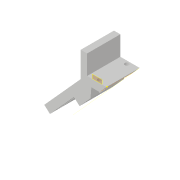
# Autodesk Inventor part: arm stop 48 degree bottom half
Saved by Autodesk Inventor 2018 (Build 220112000, 112)
## iProperties
Created: 2018-12-28
Part Number: arm stop 48 degree bottom half
Material: Generic
Document SubType Name: Modeling
Designer: ball
Density: 1 g/cm^3
Appearance: Default
Author: ball
Autodesk Inventor part; units mm, degrees
ref_plane "YZ Plane" through (0, 0, 0) normal (1, 0, 0) x (0, 1, 0)
ref_plane "XZ Plane" through (0, 0, 0) normal (0, 1, 0) x (-1, 0, 0)
ref_plane "Work Plane1" through (0, 0, 0) normal (0, 0, 1) x (1, 0, 0)
sketch "Sketch1" plane through (0, 0, 0) normal (0, 0, 1) x (1, 0, 0)
  line L0 (4.129202, -9.5377) -> (6.406797, -9.5377) construction
  line L1 (9.525, -8.41296) -> (9.525, -7.435497) construction
  line L2 (-6.406797, 9.5123) -> (-4.129202, 9.5123) construction
  line L3 (-9.525, 4.116502) -> (-9.525, 6.394097) construction
  line L4 (9.314549, -9.373063) -> (-73.965447, -101.864868) construction
  line L5 (9.166309, -9.5377) -> (-73.965447, -101.864868)
  line L6 (-73.965447, -101.864868) -> (-85.121243, -91.820144)
  line L7 (6.33881, 9.756536) -> (-85.121243, -91.820144) construction
  line L8 (9.166309, -9.5377) -> (-9.997679, -9.5377)
  line L9 (-9.997679, -9.5377) -> (-9.997679, 9.756536)
  line L10 (-9.997679, 9.756536) -> (-16.347679, 9.756536)
  line L11 (-16.347679, 9.756536) -> (-16.347679, -15.439362)
  line L12 (-16.347679, -15.439362) -> (-85.121243, -91.820144)
  point P0 (0, 0)
  dimension "d0" = 124.46
  dimension "d1" = 48
  dimension "d5" = 6.35
  constraints: 26 end point, 4 point on line, 3 horizontal, 3 perpendicular, 2 collinear, 2 vertical, 1 parallel, 8 other
  measures "d0" distance of L4.start L4.end
  measures "d1" angle of L0 L4
  measures "d5" distance of L9.end L10.end
ref_plane "Work Plane2" through (-4.445, -9.144, -33.02) normal (0, 0, -1) x (0, 1, 0)
extrude "Extrusion1" add sketch "Sketch1" against normal up to surface (33.02 mm away)
sketch "Sketch2" plane through (-73.965447, -101.864868, -33.02) normal (-0.6691306, -0.7431448, 0) x (0.7431448, -0.6691306, 0)
  line L0 (0, 33.02) -> (0, 0)
  line L1 (-15.011605, 33.02) -> (-15.011605, 0)
  line L2 (0, 0) -> (-15.011605, 0)
  line L3 (-15.011605, 0) -> (-15.011605, 26.67)
  line L4 (-15.011605, 26.67) -> (0, 26.67)
  line L5 (0, 26.67) -> (0, 0)
  line L6 (-15.011605, 33.02) -> (0, 33.02)
  point P0 (-13.193862, 33.02)
  dimension "d19" = 6.35
  constraints: 8 end point, 2 parallel, 1 horizontal, 1 perpendicular, 1 point on line
  measures "d19" distance between parallel lines of L6 L4
extrude "Extrusion2" cut sketch "Sketch2" against normal blind 25.4 contours L0 L2 L1 L4
sketch "Sketch3" plane through (-73.965447, -101.864868, -6.35) normal (0, 0, -1) x (-0.7431448, 0.6691306, 0)
  line L0 (19.8882, 12.0904) -> (19.8882, 3.175) construction
  line L1 (0, 25.4) -> (15.011605, 25.4) construction
  line L2 (15.011605, 0) -> (0, 0) construction
  line L3 (0, 0) -> (19.8882, 0) construction
  line L4 (19.8882, 0) -> (19.8882, 25.4) construction
  line L5 (19.8882, 25.4) -> (0, 25.4) construction
  line L6 (0, 25.4) -> (0, 0) construction
  line L7 (15.011605, 0) -> (19.8882, 0)
  line L8 (19.8882, 0) -> (19.8882, 25.4)
  line L9 (19.8882, 25.4) -> (15.011605, 25.4)
  line L10 (15.011605, 25.4) -> (15.011605, 0)
  point P0 (13.193862, 125.192894)
  constraints: 18 end point, 4 parallel, 2 horizontal, 2 perpendicular, 1 vertical, 2 other
extrude "Extrusion3" add sketch "Sketch3" against normal up to surface (6.35 mm away)
sketch "Sketch4" plane through (0, 0, 0) normal (0, 0, 1) x (1, 0, 0)
  line L0 (-88.74526, -88.557064) -> (-71.749342, -69.681186) construction
  line L1 (-73.965447, -101.864868) -> (9.166309, -9.5377) construction
  line L2 (-74.314967, -94.50927) -> (-67.5166, -86.958918) construction
  line L3 (-73.965447, -101.864868) -> (-56.969529, -82.988989) construction
  line L4 (-73.965447, -101.864868) -> (-88.74526, -88.557064) construction
  line L5 (-81.390199, -88.138702) -> (-74.591832, -80.588351) construction
  line L6 (-74.314967, -94.50927) -> (-67.5166, -86.958918) construction
  line L7 (-73.144662, -95.563017) -> (-66.346296, -88.012665)
  line L8 (-68.686904, -85.905171) -> (-75.485271, -93.455523)
  arc A0 (-75.485271, -93.455523) -> (-73.144662, -95.563017) centre (-74.314967, -94.50927) ccw
  arc A1 (-66.346296, -88.012665) -> (-68.686904, -85.905171) centre (-67.5166, -86.958918) ccw
  line L9 (-81.390199, -88.138702) -> (-74.591832, -80.588351) construction
  line L10 (-80.219894, -89.192449) -> (-73.421527, -81.642098)
  line L11 (-75.762136, -79.534604) -> (-82.560503, -87.084955)
  arc A2 (-82.560503, -87.084955) -> (-80.219894, -89.192449) centre (-81.390199, -88.138702) ccw
  arc A3 (-73.421527, -81.642098) -> (-75.762136, -79.534604) centre (-74.591832, -80.588351) ccw
  point P0 (0, 0)
  point P1 (-70.915783, -90.734094)
  point P2 (-77.991015, -84.363527)
  dimension "d37" = 10.16
  dimension "d38" = 5.1816
  dimension "d39" = 5.2324
  dimension "d40" = 9.52066
  dimension "d41" = 3.1496
  dimension "d42" = 3.1496
  constraints: 20 end point, 8 point on circle, 8 tangent, 4 centre point, 4 parallel, 2 collinear, 2 midpoint
  measures "d37" distance of L2.start L2.end
  measures "d38" distance between parallel lines of L1 L2
  measures "d39" distance from line of L2.start L4
  measures "d40" distance between parallel lines of L2 L5
  measures "d41" diameter of A1
  measures "d42" diameter of A3
extrude "Extrusion4" cut sketch "Sketch4" against normal through all
sketch "Sketch6" plane through (-9.997679, -9.5377, 0) normal (0, 1, 0) x (1, 0, 0)
  arc A0 (9.506526, 4.79213) -> (10.740649, 4.300966) centre (9.523849, 3.039616) ccw construction
  arc A1 (9.506526, 31.732899) -> (10.740649, 31.241734) centre (9.523849, 29.980384) ccw construction
  circle A2 centre (9.523849, 29.980384) radius 1.9685
  circle A3 centre (9.523849, 3.039616) radius 1.9685
  point P0 (9.997679, 0)
  dimension "d24" = 3.937
  dimension "d25" = 3.937
  constraints: 4 centre point, 4 point on circle, 2 coincident, 8 other
  measures "d24" diameter of A2
  measures "d25" diameter of A3
extrude "Extrusion6" cut sketch "Sketch6" against normal through all
sketch "Sketch7" plane through (9.166309, -9.5377, 0) normal (0.7431448, -0.6691306, 0) x (0, 0, -1)
  line L0 (33.02, -98.838459) -> (33.02, 0) construction
  line L1 (33.02, -9.525) -> (0, -9.525) construction
  point P0 (0, 0.954435)
  constraints: 2 end point, 1 perpendicular, 1 point on line
sketch "Sketch8" plane through (9.166309, -9.5377, -33.02) normal (0, 0, -1) x (-1, 0, 0)
  line L0 (11.608639, 0) -> (11.608639, -12.892699) construction
  line L1 (66.135838, -73.451289) -> (0, 0) construction
  line L2 (11.608639, -7.62) -> (6.861079, -7.62) construction
  line L3 (0, 0) -> (19.163987, 0) construction
  line L4 (7.671639, 0) -> (7.671639, -8.520218) construction
  line L5 (14.910639, 0) -> (14.910639, -14.251905) construction
  line L6 (6.861079, -7.62) -> (14.910639, -7.62)
  line L7 (83.131755, -92.327168) -> (0, 0)
  line L8 (15.69062, -17.426199) -> (6.861079, -7.62)
  line L9 (15.69062, -17.426199) -> (14.910639, -7.62)
  point P0 (9.166309, 9.5377)
  dimension "d28" = 7.62
  dimension "d29" = 3.302
  constraints: 10 end point, 5 point on line, 1 collinear, 1 horizontal, 1 parallel
  measures "d28" distance between parallel lines of L3 L2
  measures "d29" distance between parallel lines of L0 L5
extrude "Extrusion7" cut sketch "Sketch8" against normal blind 8.763
sketch "Sketch9" plane through (0, 0, 0) normal (0, 0, 1) x (1, 0, 0)
  line L0 (2.30523, -17.1577) -> (-5.74433, -17.1577) construction
  line L1 (-5.74433, -17.1577) -> (-6.524312, -26.963899) construction
  line L2 (2.30523, -17.1577) -> (-6.524312, -26.963899)
  line L3 (-73.965447, -101.864868) -> (9.166309, -9.5377)
  line L4 (2.30523, -17.1577) -> (-5.74433, -17.1577)
  line L5 (-5.2705, -26.963899) -> (-5.2705, -17.1577)
  point P0 (0, 0)
  constraints: 4 end point, 1 collinear, 1 vertical
sketch "Sketch9 outline for Extrusion8" plane through (0, 0, 0) normal (0, 0, 1) x (1, 0, 0)
  line L0 (-6.524312, -26.963899) -> (2.30523, -17.1577)
  line L1 (-5.74433, -17.1577) -> (-6.524312, -26.963899)
  line L2 (2.30523, -17.1577) -> (-5.74433, -17.1577)
extrude "Extrusion8" cut sketch "Sketch9 outline for Extrusion8" against normal blind 8.763
sketch "Sketch10" plane through (9.166309, -9.5377, -33.02) normal (0, 0, -1) x (-1, 0, 0)
  line L0 (25.513987, -5.901662) -> (77.291634, -63.406565)
  line L1 (67.094084, -52.081038) -> (55.938287, -62.125762)
  line L2 (66.135838, -73.451289) -> (15.69062, -17.426199) construction
  line L3 (40.913229, -45.438744) -> (36.5125, -40.551239) construction
  line L4 (66.135838, -73.451289) -> (77.291634, -63.406565) construction
  point P0 (9.166309, 9.5377)
  dimension "d34" = 15.24
  constraints: 4 end point, 3 point on line, 1 midpoint, 1 perpendicular
  measures "d34" distance between parallel lines of L1 L4
sketch "Sketch11" plane through (-73.965447, -101.864868, -6.35) normal (0, 0, -1) x (-0.7431448, 0.6691306, 0)
  arc A0 (3.6068, 5.2324) -> (6.7564, 5.2324) centre (5.1816, 5.2324) ccw construction
  arc A1 (6.7564, 15.3924) -> (3.6068, 15.3924) centre (5.1816, 15.3924) ccw construction
  line L0 (5.1816, 5.2324) -> (5.1816, 15.3924) construction
  arc A2 (13.127463, 5.2324) -> (16.277063, 5.2324) centre (14.702263, 5.2324) ccw construction
  arc A3 (16.277063, 15.3924) -> (13.127463, 15.3924) centre (14.702263, 15.3924) ccw construction
  line L1 (14.702263, 5.2324) -> (14.702263, 15.3924) construction
  line L2 (14.702263, 5.2324) -> (14.702263, 15.3924) construction
  line L3 (17.877263, 5.2324) -> (17.877263, 15.3924)
  line L4 (11.527263, 15.3924) -> (11.527263, 5.2324)
  arc A4 (11.527263, 5.2324) -> (17.877263, 5.2324) centre (14.702263, 5.2324) ccw
  arc A5 (17.877263, 15.3924) -> (11.527263, 15.3924) centre (14.702263, 15.3924) ccw
  line L5 (5.1816, 5.2324) -> (5.1816, 15.3924) construction
  line L6 (8.3566, 5.2324) -> (8.3566, 15.3924)
  line L7 (2.0066, 15.3924) -> (2.0066, 5.2324)
  arc A6 (2.0066, 5.2324) -> (8.3566, 5.2324) centre (5.1816, 5.2324) ccw
  arc A7 (8.3566, 15.3924) -> (2.0066, 15.3924) centre (5.1816, 15.3924) ccw
  point P0 (13.193862, 125.192894)
  point P1 (14.702263, 10.3124)
  point P2 (5.1816, 10.3124)
  dimension "d43" = 6.35
  dimension "d44" = 6.35
  constraints: 20 end point, 8 point on circle, 8 tangent, 4 centre point, 4 equal length, 2 midpoint, 2 vertical
  measures "d43" diameter of A5
  measures "d44" diameter of A7
extrude "Extrusion9" cut sketch "Sketch11" against normal blind 3.556
split body "Split1" sketch "Sketch10" result one side removed curves L1 removed pieces at (-50.542289, -75.103577, -13.123333)
sketch "Sketch13" plane through (9.166309, -9.5377, -33.02) normal (0, 0, -1) x (-1, 0, 0)
  line L0 (55.938287, -62.125762) -> (15.69062, -17.426199)
  line L1 (55.938287, -62.125762) -> (67.094084, -52.081038)
  line L2 (55.938287, -62.125762) -> (50.414614, -55.991102)
  line L3 (50.414614, -55.991102) -> (61.570411, -45.946377)
  line L4 (61.570411, -45.946377) -> (67.094084, -52.081038)
  line L5 (67.094084, -52.081038) -> (55.938287, -62.125762)
  point P0 (9.166309, 9.5377)
  dimension "d48" = 8.255
  constraints: 8 end point, 2 parallel, 1 perpendicular, 1 point on line
  measures "d48" distance between parallel lines of L3 L1
extrude "Extrusion10" cut sketch "Sketch13" against normal through all
sketch "Sketch15" plane through (9.166309, -9.5377, 0) normal (0.7431448, -0.6691306, 0) x (0, 0, -1)
  line L0 (7.62, -71.533459) -> (7.62, -44.863459) construction
  line L1 (0, -75.343459) -> (0, -23.449264) construction
  line L2 (0, -75.343459) -> (33.02, -75.343459) construction
  line L3 (25.4, -71.533459) -> (25.4, -44.863459) construction
  line L4 (33.02, -75.343459) -> (33.02, -23.449264) construction
  line L5 (7.62, -71.533459) -> (7.62, -44.863459) construction
  line L6 (9.5885, -71.533459) -> (9.5885, -44.863459)
  line L7 (5.6515, -44.863459) -> (5.6515, -71.533459)
  arc A0 (5.6515, -71.533459) -> (9.5885, -71.533459) centre (7.62, -71.533459) ccw
  arc A1 (9.5885, -44.863459) -> (5.6515, -44.863459) centre (7.62, -44.863459) ccw
  line L8 (25.4, -71.533459) -> (25.4, -44.863459) construction
  line L9 (27.3685, -71.533459) -> (27.3685, -44.863459)
  line L10 (23.4315, -44.863459) -> (23.4315, -71.533459)
  arc A2 (23.4315, -71.533459) -> (27.3685, -71.533459) centre (25.4, -71.533459) ccw
  arc A3 (27.3685, -44.863459) -> (23.4315, -44.863459) centre (25.4, -44.863459) ccw
  point P0 (0, 0.954435)
  point P1 (7.62, -58.198459)
  point P2 (25.4, -58.198459)
  dimension "d51" = 7.62
  dimension "d52" = 3.81
  dimension "d53" = 7.62
  dimension "d54" = 30.48
  dimension "d55" = 3.81
  dimension "d56" = 30.48
  dimension "d57" = 3.937
  dimension "d58" = 3.937
  constraints: 20 end point, 8 point on circle, 8 tangent, 4 centre point, 3 parallel, 2 midpoint, 1 collinear, 1 vertical
  measures "d51" distance between parallel lines of L1 L0
  measures "d52" distance from line of L2 L0.start
  measures "d53" distance between parallel lines of L4 L3
  measures "d54" distance from line of L2 L0.end
  measures "d55" vertical distance of L2.end L3.start
  measures "d56" distance from line of L2 L3.end
  measures "d57" diameter of A1
  measures "d58" diameter of A3
extrude "Extrusion11" cut sketch "Sketch15" against normal through all
sketch "Sketch16" plane through (9.166309, -9.5377, -33.02) normal (0, 0, -1) x (-1, 0, 0)
  line L0 (50.414614, -55.991102) -> (15.69062, -17.426199)
  line L1 (50.414614, -55.991102) -> (26.62033, -29.564872)
  line L2 (26.62033, -29.564872) -> (32.198152, -24.542578)
  line L3 (32.198152, -24.542578) -> (55.992436, -50.968808)
  line L4 (55.992436, -50.968808) -> (50.414614, -55.991102)
  point P0 (9.166309, 9.5377)
  dimension "d61" = 35.56
  dimension "d62" = 7.5057
  constraints: 8 end point, 2 parallel, 1 perpendicular, 1 point on line
  measures "d61" distance between parallel lines of L2 L4
  measures "d62" distance between parallel lines of L0 L3
extrude "Extrusion12" cut sketch "Sketch16" against normal through all
body "Solid1"
